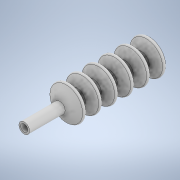
# Autodesk Inventor part: linear_actuator_test
Saved by Autodesk Inventor 2021 (Build 250183000, 183)
## iProperties
Created: 2021-05-06
Part Number: linear_actuator_test
Material: Generic
Document SubType Name: Modeling
Designer: Charlie
Density: 1 g/cm^3
Appearance: Default
Author: Charlie
Autodesk Inventor part; units mm, degrees
ref_plane "YZ Plane" through (0, 0, 0) normal (1, 0, 0) x (0, 1, 0)
ref_plane "XY Plane" through (0, 0, 0) normal (0, 0, 1) x (1, 0, 0)
sketch "Sketch1" plane through (0, 0, 0) normal (0, 1, 0) x (-1, 0, 0)
  line L0 (0, 0) -> (-9, 0)
  line L1 (0, 0) -> (0, -9) construction
  line L2 (1, 0) -> (7.2029, -3.6374)
  line L3 (7.2029, -5.3626) -> (2.4711, -8.1374)
  line L4 (2.4711, -9.8626) -> (7.2029, -12.6374)
  line L5 (7.2029, -14.3626) -> (2.4711, -17.1374)
  line L6 (2.4711, -18.8626) -> (7.2029, -21.6374)
  line L7 (7.2029, -23.3626) -> (2.4711, -26.1374)
  line L8 (2.4711, -27.8626) -> (7.2029, -30.6374)
  line L9 (7.2029, -32.3626) -> (2.4711, -35.1374)
  line L10 (2.4711, -36.8626) -> (7.2029, -39.6374)
  line L11 (7.2029, -41.3626) -> (2.4711, -44.1374)
  line L12 (2.4711, -45.8626) -> (7.2029, -48.6374)
  line L13 (7.2029, -50.3626) -> (1, -54)
  line L14 (1, -54) -> (-2, -54)
  line L15 (0, 0) -> (-2, 0)
  line L16 (-2, 0) -> (-2, -54)
  arc A0 (7.2029, -5.3626) -> (7.2029, -3.6374) centre (6.697, -4.5) ccw
  arc A1 (7.2029, -14.3626) -> (7.2029, -12.6374) centre (6.697, -13.5) ccw
  arc A2 (7.2029, -23.3626) -> (7.2029, -21.6374) centre (6.697, -22.5) ccw
  arc A3 (7.2029, -32.3626) -> (7.2029, -30.6374) centre (6.697, -31.5) ccw
  arc A4 (7.2029, -41.3626) -> (7.2029, -39.6374) centre (6.697, -40.5) ccw
  arc A5 (7.2029, -50.3626) -> (7.2029, -48.6374) centre (6.697, -49.5) ccw
  line L17 (1, 20) -> (0, 20) construction
  line L18 (0, 0) -> (0, 20) construction
  line L19 (-2, 0) -> (-2, 20)
  line L20 (-2, 20) -> (1, 20)
  line L21 (1, 0) -> (1, 20)
  arc A6 (2.4711, -8.1374) -> (2.4711, -9.8626) centre (2.9769, -9) ccw
  arc A7 (2.4711, -17.1374) -> (2.4711, -18.8626) centre (2.9769, -18) ccw
  arc A8 (2.4711, -26.1374) -> (2.4711, -27.8626) centre (2.9769, -27) ccw
  arc A9 (2.4711, -35.1374) -> (2.4711, -36.8626) centre (2.9769, -36) ccw
  arc A10 (2.4711, -44.1374) -> (2.4711, -45.8626) centre (2.9769, -45) ccw
  point P0 (1, -9)
  point P1 (8.6739, -4.5)
  point P2 (1, -9)
  point P3 (1, -18)
  point P4 (8.6739, -13.5)
  point P5 (1, -18)
  point P6 (1, -27)
  point P7 (8.6739, -22.5)
  point P8 (1, -27)
  point P9 (8.6739, -31.5)
  point P10 (1, -36)
  point P11 (1, -36)
  point P12 (1, -45)
  point P13 (8.6739, -40.5)
  point P14 (1, -45)
  point P15 (8.6739, -49.5)
  point P16 (1, -45)
  point P17 (1, -36)
  point P18 (1, -27)
  point P19 (1, -18)
  point P20 (1, -9)
  point P21 (1, 0)
  dimension "d1" = 9
  dimension "d2" = 7.6739
  dimension "d3" = 120.387
  dimension "d4" = 9
  dimension "d5" = 7.6739
  dimension "d6" = 9
  dimension "d7" = 7.6739
  dimension "d8" = 9
  dimension "d9" = 7.6739
  dimension "d10" = 9
  dimension "d11" = 7.6739
  dimension "d12" = 9
  dimension "d13" = 7.6739
  dimension "d15" = 2
  dimension "d16" = 1
  dimension "d19" = 1
  dimension "d20" = 20
  dimension "d23" = 1
  constraints: 45 end point, 23 point on line, 22 point on circle, 22 tangent, 11 centre point, 9 equal radius, 3 perpendicular, 2 horizontal, 2 vertical
  measures "d1" distance of L1.end L0.start
  measures "d2" horizontal distance of point (8.674, -4.5) point (1, -9)
  measures "d3" angle of L2 L1
  measures "d4" distance of point (1, -9) point (1, -18)
  measures "d5" horizontal distance of point (8.674, -13.5) point (1, -18)
  measures "d6" distance of point (1, -18) point (1, -27)
  measures "d7" horizontal distance of point (8.674, -22.5) point (1, -27)
  measures "d8" distance of point (1, -27) point (1, -36)
  measures "d9" horizontal distance of point (8.674, -31.5) point (1, -36)
  measures "d10" distance of point (1, -36) point (1, -45)
  measures "d11" horizontal distance of point (8.674, -40.5) point (1, -45)
  measures "d12" distance of L13.end point (1, -45)
  measures "d13" horizontal distance of L13.end point (8.674, -49.5)
  measures "d15" distance of L0.start L15.end
  measures "d16" radius of A0
  measures "d19" distance of L17.start L17.end
  measures "d20" distance of L0.start L17.end
  measures "d23" radius of A6
revolve "Revolution1" add sketch "Sketch1" angle 360 about axis through (2, 0, 0) along (0, 0, -1)
shell "Shell1" thickness 1 removed faces 1 at (1.071, 0.823, 20)
sketch "Sketch3" plane through (0, 0, 0) normal (0, 1, 0) x (-1, 0, 0)
  line L0 (12.3596, 25.7411) -> (-16.3497, 25.7411)
  line L1 (-16.3497, 25.7411) -> (-16.3497, -59.9976)
  line L2 (-16.3497, -59.9976) -> (12.3596, -59.9976)
  line L3 (12.3596, -59.9976) -> (12.3596, 25.7411)
  point P0 (0, 0)
  constraints: 8 end point, 2 parallel, 1 horizontal, 1 perpendicular
body "Solid1"
